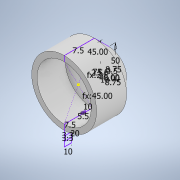
# Autodesk Inventor part: AirFeed1
Saved by Autodesk Inventor 2020.1 (Build 241239000, 239)
## iProperties
Created: 2019-11-11
Part Number: AirFeed1
Material: Generic
Document SubType Name: Modeling
Designer: Paul Lefeuvre
Density: 1 g/cm^3
Appearance: Default
Author: Paul Lefeuvre
Autodesk Inventor part; units mm, degrees
ref_plane "YZ Plane" through (0, 0, 0) normal (1, 0, 0) x (0, 1, 0)
ref_plane "XZ Plane" through (0, 0, 0) normal (0, 1, 0) x (-1, 0, 0)
ref_plane "XY Plane" through (0, 0, 0) normal (0, 0, 1) x (1, 0, 0)
sketch "Sketch1" plane through (0, 0, 0) normal (1, 0, 0) x (0, 1, 0)
  line L0 (37.8, 19.7) -> (37.8, -19.7)
  line L1 (37.8, -19.7) -> (-37.8, -19.7)
  line L2 (-37.8, -19.7) -> (-37.8, 19.7)
  line L3 (-37.8, 19.7) -> (37.8, -19.7) construction
  line L4 (37.8, 19.7) -> (-37.8, -19.7) construction
  line L5 (45.3, -22.2981) -> (45.3, 19.7)
  line L6 (-45.3, 9.7) -> (-45.3, -22.2981)
  line L7 (-45.3, -22.2981) -> (-25, -42.5981)
  line L8 (25, -42.5981) -> (45.3, -22.2981)
  line L9 (0, -42.5981) -> (0, -19.7) construction
  line L10 (-2.5, -19.7) -> (-2.5, -42.5981)
  line L11 (2.5, -19.7) -> (2.5, -42.5981)
  line L12 (37.8, 19.7) -> (45.3, 19.7)
  line L13 (-37.8, 19.7) -> (-45.3, 19.7)
  line L14 (25, -42.5981) -> (-25, -42.5981)
  line L15 (-45.3, 19.7) -> (-65.3, 19.7)
  line L16 (-65.3, 19.7) -> (-65.3, 9.7)
  line L17 (-65.3, 9.7) -> (-45.3, 9.7)
  line L18 (-45.3, 9.7) -> (-45.3, 19.7)
  line L19 (-55.3, 9.7) -> (-55.3, 19.7) construction
  line L20 (-52, 9.7) -> (-52, 19.7)
  line L21 (-58.6, 9.7) -> (-58.6, 19.7)
  line L22 (37.8, -19.7) -> (24.9019, -32.5981)
  line L23 (24.9019, -32.5981) -> (-24.9019, -32.5981)
  line L24 (-24.9019, -32.5981) -> (-37.8, -19.7)
  line L25 (-37.8, -9.7) -> (-45.3, -9.7)
  line L26 (-37.8, -4.2) -> (-45.3, -4.2)
  line L27 (-16.25, -42.5981) -> (-14.133, -45.1211)
  line L28 (-13.367, -45.1211) -> (-11.25, -42.5981)
  line L29 (-13.75, -45.5775) -> (-13.75, -42.5981)
  arc A0 (-14.133, -45.1211) -> (-13.367, -45.1211) centre (-13.75, -44.7997) ccw
  line L30 (-45.3, -4.2) -> (-49.2679, -4.2)
  line L31 (-49.2679, -4.2) -> (-49.2679, -9.7)
  line L32 (-49.2679, -9.7) -> (-45.3, -9.7)
  line L33 (-45.3, -9.7) -> (-45.3, -4.2)
  line L34 (-37.8, -9.7) -> (-35.6773, -9.7)
  line L35 (-35.6773, -9.7) -> (-35.6773, -4.2)
  line L36 (-35.6773, -4.2) -> (-37.8, -4.2)
  line L37 (-37.8, -4.2) -> (-37.8, -9.7)
  line L38 (-49.2679, -6.95) -> (-35.6773, -6.95)
  point P0 (0, 0)
  point P1 (2.5, -32.5981)
  point P2 (-2.5, -32.5981)
  point P3 (-13.75, -45.2997)
  dimension "d0" = 75.6
  dimension "d2" = 7.5
  dimension "d3" = 45
  dimension "d4" = 45
  dimension "d5" = 7.5
  dimension "d7" = 2.5
  dimension "d8" = 2.5
  dimension "d9" = 50
  dimension "d17" = 20
  dimension "d18" = 10
  dimension "d19" = 3.3
  dimension "d20" = 3.3
  dimension "d22" = 10
  dimension "d23" = 5.5
  dimension "d24" = 10
  dimension "d30" = 8.75
  dimension "d31" = 8.75
  dimension "d32" = 40
  dimension "d33" = 40
  dimension "d34" = 0.5
  constraints: 76 end point, 13 parallel, 10 point on line, 8 perpendicular, 7 midpoint, 4 horizontal, 2 point on circle, 2 tangent, 2 vertical, 1 centre point, 10 other
  measures "d0" distance of L0.end L1.end
  measures "d2" distance between parallel lines of L0 L5
  measures "d3" angle of L1 L8
  measures "d4" angle of L1 L7
  measures "d5" distance between parallel lines of L2 L6
  measures "d7" distance between parallel lines of L11 L9
  measures "d8" distance between parallel lines of L9 L10
  measures "d9" distance of L7.end L8.start
  measures "d17" distance of L16.end L6.start
  measures "d18" distance of L15.end L16.end
  measures "d19" distance between parallel lines of L19 L20
  measures "d20" distance between parallel lines of L19 L21
  measures "d23" distance between parallel lines of L25 L26
  measures "d24" distance of L25.start L1.end
  measures "d30" distance of L7.end L27.start
  measures "d31" distance of L10.end L28.end
  measures "d32" angle of L28 L29
  measures "d33" angle of L29 L27
  measures "d34" radius of A0
revolve "Revolution1" add sketch "Sketch1" angle 360 about axis through (0, 0, -42.5981) along (0, 0, 1) contours L12 L5 L8 L14 L11 L23 L22 L0 | L24 L23 L10 L14 L7 L6 L25 L2 | L25 L6 L38 L2 | L38 L6 L26 L2 | L26 L6 L18 L13 L2
revolve "Revolution2" add sketch "Sketch1" angle 360 about axis through (0, -13.75, -45.5775) along (0, 0, 1) contours L28 A0 L29 L14
revolve "Revolution3" cut sketch "Sketch1" angle 360 about axis through (0, -49.2679, -6.95) along (0, 1, 0) contours L38 L6 L26 L2 | L2 L36 L35 L38 | L38 L31 L30 L6
equation "\"d4\" = d3"
equation "\"d8\" = d7"
body "Solid1"
